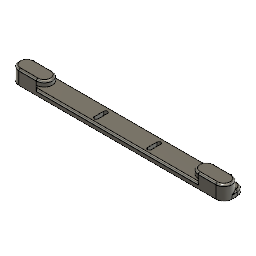
HeatedBedHolderV2 (Autodesk Fusion 360 design; units mm, degrees)
Autodesk Fusion 360 part; units mm, degrees
sketch "Sketch1" plane through (0, 0, 0) normal (0, 1, 0) x (1, 0, 0)
  line L0 (100, 0) -> (24, 0)
  line L1 (100, 0) -> (176, 0)
  line L2 (176, 0) -> (224, 0) construction
  arc A0 (24, 0) -> (24, 15) centre (24, 7.5) ccw
  arc A1 (176, 15) -> (176, 0) centre (176, 7.5) ccw
  arc A2 (7.5, 15) -> (7.5, 0) centre (7.5, 7.5) ccw
  arc A3 (192.5, 0) -> (192.5, 15) centre (192.5, 7.5) ccw
  arc A4 (7.5, 25) -> (0, 17.5) centre (7.5, 17.5) ccw
  arc A5 (200, 17.5) -> (192.5, 25) centre (192.5, 17.5) ccw
  line L3 (9.5662, 25) -> (12.453, 20)
  line L4 (192.5, 25) -> (190.4338, 25)
  line L5 (190.4338, 25) -> (187.547, 20)
  line L6 (187.547, 20) -> (12.453, 20)
  line L7 (7.5, 25) -> (9.5662, 25)
  line L8 (192.5, 0) -> (7.5, 0)
  line L9 (0, 17.5) -> (0, 7.5)
  line L10 (200, 17.5) -> (200, 7.5)
  line L11 (100, 20) -> (100, 0)
  line L12 (123.25, 15.0004) -> (123.25, 4)
  line L13 (126.75, 15.0004) -> (126.75, 4)
  arc A6 (126.75, 15.0004) -> (123.25, 15.0004) centre (125, 15) ccw
  arc A7 (123.25, 4) -> (126.75, 4) centre (125, 4) ccw
  line L14 (73.25, 15.0004) -> (73.25, 4)
  arc A8 (76.75, 15.0004) -> (73.25, 15.0004) centre (75, 15) ccw
  line L15 (76.75, 15.0004) -> (76.75, 4)
  arc A9 (73.25, 4) -> (76.75, 4) centre (75, 4) ccw
  line L16 (24, 0) -> (12.453, 20)
  line L17 (176, 0) -> (187.547, 20)
  line L18 (176, 15) -> (192.5, 15)
  line L19 (7.5, 15) -> (24, 15)
  point P0 (7.5, 17.5)
  point P1 (192.5, 17.5)
extrude "Extrude1" add sketch "Sketch1" against normal blind 5 makes body 1
extrude "Extrude2" add sketch "Sketch1" along normal blind 5 contours A0 L16 L19 | A2 L8 L16 L19 | A3 L8 L17 L18 | A1 L17 L18 | A2 A4 L3 L7 L9 L16 L19 | A3 A5 L4 L5 L10 L17 L18 bodies 1
extrude "Extrude3" add sketch "Sketch1" along normal blind 10 separate body contours A0 L16 L19 | A2 L8 L16 L19 | A3 L8 L17 L18 | A1 L17 L18 makes body 2 at (18.5, 0, -5) makes body 3 at (187, 0, -5)
extrude "Extrude4" cut sketch "Sketch1" along normal blind 3.5 contours A0 L16 L19 | A1 L17 L18 bodies 2 3
extrude "Extrude5" cut 2 faces at (187, 10, -5) (18.5, 10, -5) along direction (0, -1, 0) blind 1.5 on bodies 2 3 bodies 2 3
extrude "Extrude6" cut 2 faces at (184.3868, 5, -5) (15.6132, 5, -5) along direction (0, -1, 0) blind 5 on bodies 1 bodies 1
combine "Combine1" operation add target body 3 tool bodies 2 1
sketch "Sketch2" plane through (0, 0, 0) normal (0, 1, 0) x (-1, 0, 0)
  arc A0 (-76.75, -15.0004) -> (-73.25, -15.0004) centre (-75, -15) ccw
  line L0 (-76.75, -15.0004) -> (-76.75, -4)
  arc A1 (-73.25, -4) -> (-76.75, -4) centre (-75, -4) ccw
  line L1 (-73.25, -4) -> (-73.25, -15.0004)
  arc A2 (-126.75, -15.0004) -> (-123.25, -15.0004) centre (-125, -15) ccw
  line L2 (-126.75, -15.0004) -> (-126.75, -4)
  arc A3 (-123.25, -4) -> (-126.75, -4) centre (-125, -4) ccw
  line L3 (-123.25, -4) -> (-123.25, -15.0004)
  line L4 (-176, 0) -> (-184.6603, -15)
  line L5 (-184.6603, -15) -> (-192.5, -15)
  arc A4 (-200, -7.5) -> (-192.5, -15) centre (-192.5, -7.5) ccw
  line L6 (-200, -7.5) -> (-200, -17.5)
  arc A5 (-200, -17.5) -> (-192.5, -25) centre (-192.5, -17.5) ccw
  line L7 (-192.5, -25) -> (-190.4338, -25)
  line L8 (-190.4338, -25) -> (-187.547, -20)
  line L9 (-187.547, -20) -> (-12.453, -20)
  line L10 (-12.453, -20) -> (-9.5662, -25)
  line L11 (-9.5662, -25) -> (-7.5, -25)
  arc A6 (-7.5, -25) -> (0, -17.5) centre (-7.5, -17.5) ccw
  line L12 (0, -17.5) -> (0, -7.5)
  arc A7 (-7.5, -15) -> (0, -7.5) centre (-7.5, -7.5) ccw
  line L13 (-7.5, -15) -> (-15.3397, -15)
  line L14 (-15.3397, -15) -> (-24, 0)
  line L15 (-24, 0) -> (-176, 0)
  arc A8 (-76.75, -14.0004) -> (-73.25, -14.0004) centre (-75, -14) ccw
  arc A9 (-73.25, -5) -> (-76.75, -5) centre (-75, -5) ccw
  line L16 (-73.25, -14.0004) -> (-73.25, -5)
  line L17 (-76.75, -5) -> (-76.75, -14.0004)
  line L18 (-100, -20) -> (-100, 0)
  line L19 (-126.75, -4) -> (-126.75, -15.0004)
  line L20 (-123.25, -15.0004) -> (-123.25, -4)
  arc A10 (-126.75, -14.0004) -> (-123.25, -14.0004) centre (-125, -14) ccw
  arc A11 (-123.25, -5) -> (-126.75, -5) centre (-125, -5) ccw
  line L21 (-123.25, -5) -> (-123.25, -14.0004)
  line L22 (-126.75, -14.0004) -> (-126.75, -5)
  point P0 (-125, -4)
  point P1 (-125, -15)
extrude "Extrude7" add sketch "Sketch2" against normal blind 5 contours A0 L0 L1 A8 | L0 A1 L1 A9 | A2 L2 L3 L19 L20 A10 | L2 A3 L3 L19 L20 A11 bodies 3
sketch "Sketch3" plane through (0, 0, 0) normal (0, 1, 0) x (-1, 0, 0)
  arc A0 (-76.75, -14.0004) -> (-73.25, -14.0004) centre (-75, -14) ccw
  line L0 (-76.75, -14.0004) -> (-76.75, -5)
  arc A1 (-73.25, -5) -> (-76.75, -5) centre (-75, -5) ccw
  line L1 (-73.25, -5) -> (-73.25, -14.0004)
  arc A2 (-126.75, -14.0004) -> (-123.25, -14.0004) centre (-125, -14) ccw
  line L2 (-126.75, -14.0004) -> (-126.75, -5)
  arc A3 (-123.25, -5) -> (-126.75, -5) centre (-125, -5) ccw
  line L3 (-123.25, -5) -> (-123.25, -14.0004)
  line L4 (-176, 0) -> (-184.6603, -15)
  line L5 (-184.6603, -15) -> (-192.5, -15)
  arc A4 (-200, -7.5) -> (-192.5, -15) centre (-192.5, -7.5) ccw
  line L6 (-200, -7.5) -> (-200, -17.5)
  arc A5 (-200, -17.5) -> (-192.5, -25) centre (-192.5, -17.5) ccw
  line L7 (-192.5, -25) -> (-190.4338, -25)
  line L8 (-190.4338, -25) -> (-187.547, -20)
  line L9 (-187.547, -20) -> (-12.453, -20)
  line L10 (-12.453, -20) -> (-9.5662, -25)
  line L11 (-9.5662, -25) -> (-7.5, -25)
  arc A6 (-7.5, -25) -> (0, -17.5) centre (-7.5, -17.5) ccw
  line L12 (0, -17.5) -> (0, -7.5)
  arc A7 (-7.5, -15) -> (0, -7.5) centre (-7.5, -7.5) ccw
  line L13 (-7.5, -15) -> (-15.3397, -15)
  line L14 (-15.3397, -15) -> (-24, 0)
  line L15 (-24, 0) -> (-176, 0)
  arc A8 (-7.5, -20) -> (0, -12.5) centre (-7.5, -12.5) ccw
  arc A9 (-200, -12.5) -> (-192.5, -20) centre (-192.5, -12.5) ccw
  line L16 (-192.5, -20) -> (-187.547, -20)
  line L17 (-7.5, -20) -> (-12.453, -20)
extrude "Extrude8" cut sketch "Sketch3" against normal blind 5 contours L6 A5 L7 L8 A9 L16 | L10 L11 A6 L12 A8 L17 bodies 3
fillet "Fillet1" radius 1.6 14 edges at (100, 0, 0) (200, 0, -10) (197.8033, 0, -17.8033) (100, 0, -20) (2.1967, 0, -17.8033) (0, 0, -10) (0, 8.5, -7.5) (15.75, 8.5, -15) (31.5, 8.5, -7.5) (15.75, 8.5, 0) (184.25, 8.5, -15) (200, 8.5, -7.5) (184.25, 8.5, 0) (168.5, 8.5, -7.5) on bodies 3
